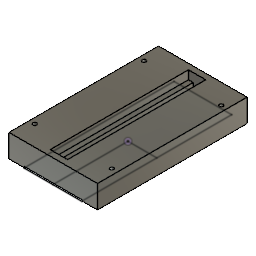
532nm_laser_mount (Autodesk Fusion 360 design; units mm, degrees)
Autodesk Fusion 360 part; units mm, degrees
note: some values were not read from the file. Set by a fixed rule: the direction of a hole.
sketch "Sketch1" plane through (0, 0, 0) normal (0, 0, 1) x (1, 0, 0)
  line L0 (-38.5, 65) -> (38.5, 65)
  line L1 (38.5, 65) -> (38.5, -65)
  line L2 (38.5, -65) -> (-38.5, -65)
  line L3 (-38.5, -65) -> (-38.5, 65)
  line L4 (0, 65) -> (0, 0)
  line L5 (0, 0) -> (38.5, 0)
  line L6 (-33.5, -47.5) -> (-33.5, -65)
  line L7 (-33.5, -47.5) -> (-38.5, -47.5)
  line L8 (-33.5, 47.5) -> (-33.5, 65)
  line L9 (-33.5, 47.5) -> (-38.5, 47.5)
  line L10 (33.5, 47.5) -> (38.5, 47.5)
  line L11 (33.5, 47.5) -> (33.5, 65)
  line L12 (33.5, -47.5) -> (38.5, -47.5)
  line L13 (33.5, -47.5) -> (33.5, -65)
  point P0 (-33.5, 47.5)
  point P1 (33.5, 47.5)
  point P2 (33.5, -47.5)
  point P3 (-33.5, -47.5)
  dimension "d2" = 77
  dimension "d3" = 130
  dimension "d21" = 5
  dimension "d22" = 17.5
  constraint horizontal L0
  constraint vertical L1
  constraint horizontal L2
  constraint vertical L3
  constraint midpoint L0 L4.start
  constraint coincident L4.end L5.start
  constraint perpendicular L0 L4
  constraint midpoint L1 L5.end
  constraint perpendicular L1 L5
  constraint coincident P3 L6.start
  constraint coincident L2 L6.end
  constraint perpendicular L2 L6
  constraint coincident L3 L7.end
  constraint perpendicular L3 L7
  constraint coincident P0 L8.start
  constraint coincident L0 L8.end
  constraint perpendicular L0 L8
  constraint coincident L3 L9.end
  constraint perpendicular L3 L9
  constraint coincident P1 L10.start
  constraint coincident L1 L10.end
  constraint perpendicular L1 L10
  constraint coincident L0 L11.end
  constraint perpendicular L0 L11
  constraint coincident P2 L12.start
  constraint coincident L1 L12.end
  constraint perpendicular L1 L12
  constraint coincident L2 L13.end
  constraint perpendicular L2 L13
  constraint equal L6 L13
  constraint equal L8 L13
  constraint equal L11 L13
  constraint equal L10 L12
  constraint equal L7 L12
  constraint equal L9 L12
  measures "d2" distance of L0.start L0.end
  measures "d3" distance of L0.end L1.end
  measures "d21" distance of P2 L12.end
  measures "d22" distance of P2 L13.end
extrude "Extrude1" add sketch "Sketch1" along normal blind 20
hole "Hole1" at (-33.5, 47.5, 0) at (33.5, 47.5, 0) at (-33.5, -47.5, 0) at (33.5, -47.5, 0) direction (0, 0, 1) diameter 3.3 end through all
sketch "Sketch2" plane through (0, 0, 20) normal (0, 0, 1) x (-1, 0, 0)
  circle A0 centre (33.5, 47.5) radius 1.65
  circle A1 centre (33.5, -47.5) radius 1.65
  circle A2 centre (-33.5, -47.5) radius 1.65
  circle A3 centre (-33.5, 47.5) radius 1.65
  line L0 (38.5, 65) -> (-38.5, 65)
  line L1 (-38.5, 65) -> (-38.5, -65)
  line L2 (-38.5, -65) -> (38.5, -65)
  line L3 (38.5, -65) -> (38.5, 65)
  line L4 (0, 0) -> (-7.5, 0)
  line L5 (0, 0) -> (0, -60)
  line L6 (7.5, -60) -> (-7.5, -60)
  line L7 (-7.5, -60) -> (-7.5, 60)
  line L8 (-7.5, 60) -> (7.5, 60)
  line L9 (7.5, 60) -> (7.5, -60)
  dimension "d12" = 15
  dimension "d13" = 120
  constraint coincident L4.start L5.start
  constraint horizontal L4
  constraint perpendicular L4 L5
  constraint horizontal L6
  constraint vertical L7
  constraint horizontal L8
  constraint vertical L9
  constraint coincident L4.end L7
  constraint midpoint L5.end L6
  constraint midpoint L4.end L7
  measures "d12" distance of L6.start L6.end
  measures "d13" distance of L6.end L7.end
extrude "Extrude2" cut sketch "Sketch2" against normal blind 7.5 contours L4 L5 L6 L7 | L4 L5 L6 L7 L8 L9
sketch "Sketch3" plane through (0, 0, 12.5) normal (0, 0, 1) x (-1, 0, 0)
  line L0 (7.5, 60) -> (-7.5, 60)
  line L1 (-7.5, 60) -> (-7.5, -60)
  line L2 (-7.5, -60) -> (7.5, -60)
  line L3 (7.5, -60) -> (7.5, 60)
  line L4 (0, 0) -> (0, -60)
  line L5 (0, 0) -> (-3.375, 0)
  line L6 (3.375, -60) -> (-3.375, -60)
  line L7 (-3.375, -60) -> (-3.375, 60)
  line L8 (-3.375, 60) -> (3.375, 60)
  line L9 (3.375, 60) -> (3.375, -60)
  dimension "d16" = 120
  dimension "d17" = 6.75
  constraint coincident L4.start L5.start
  constraint vertical L4
  constraint perpendicular L4 L5
  constraint horizontal L6
  constraint vertical L7
  constraint horizontal L8
  constraint vertical L9
  constraint midpoint L5.end L7
  constraint midpoint L4.end L6
  measures "d16" distance of L6.end L7.end
  measures "d17" distance of L6.start L6.end
extrude "Extrude3" cut sketch "Sketch3" against normal through all contours L0 L2 L4 L5 L6 L7 L8 L9 | L2 L4 L5 L6 L7
sketch "Sketch4" plane through (0, 0, 0) normal (0, 0, 1) x (1, 0, 0)
  line L0 (0, 0) -> (25, 0)
  line L1 (0, 0) -> (0, -65)
  line L2 (-25, -65) -> (25, -65)
  line L3 (25, -65) -> (25, 65)
  line L4 (25, 65) -> (-25, 65)
  line L5 (-25, 65) -> (-25, -65)
  dimension "d23" = 130
  dimension "d26" = 50
  constraint coincident L0.start L1.start
  constraint horizontal L0
  constraint perpendicular L0 L1
  constraint horizontal L2
  constraint vertical L3
  constraint horizontal L4
  constraint vertical L5
  constraint midpoint L0.end L3
  constraint midpoint L1.end L2
  measures "d23" distance of L2.end L3.end
  measures "d26" distance of L2.start L2.end
extrude "Extrude5" cut sketch "Sketch4" along normal blind 1
extrude "Extrude4" [suppressed]
